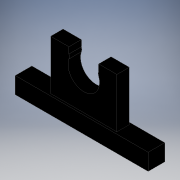
# Autodesk Inventor part: OpticalDeviceLensHolder
Saved by Autodesk Inventor 2017 (Build 210142000, 142)
## iProperties
Created: 2019-04-03
Part Number: OpticalDeviceLensHolder
Material: Generic
Document SubType Name: Modeling
Designer: Sharat
Density: 1 g/cm^3
Appearance: Anodized - Black
Author: Sharat
Autodesk Inventor part; units mm, degrees
ref_plane "YZ Plane" through (0, 0, 0) normal (1, 0, 0) x (0, 1, 0)
ref_plane "XZ Plane" through (0, 0, 0) normal (0, 1, 0) x (-1, 0, 0)
ref_plane "XY Plane" through (0, 0, 0) normal (0, 0, 1) x (1, 0, 0)
sketch "Sketch1" plane through (0, 0, 0) normal (0, 1, 0) x (-1, 0, 0)
  line L0 (0, 0) -> (-160.48, 0)
  line L1 (-160.48, 0) -> (-160.48, -20)
  line L2 (-160.48, -20) -> (0, -20)
  line L3 (0, -20) -> (0, 0)
  dimension "d0" = 160.48
  dimension "d1" = 20
  constraints: 8 end point, 2 parallel, 1 horizontal, 1 perpendicular
  measures "d0" distance of L1.end L2.end
  measures "d1" distance of L2.end L0.start
extrude "Extrusion1" add sketch "Sketch1" along normal blind 20
sketch "Sketch2" plane through (0, 20, 0) normal (0, 1, 0) x (1, 0, 0)
  line L0 (40.24, 17.5) -> (120.24, 17.5)
  line L1 (120.24, 17.5) -> (120.24, 2.5)
  line L2 (120.24, 2.5) -> (40.24, 2.5)
  line L3 (40.24, 2.5) -> (40.24, 17.5)
  line L4 (160.48, 20) -> (0, 20) projected
  line L5 (160.48, 0) -> (160.48, 20) projected
  point P0 (0, 0)
  point P1 (80.24, 17.5)
  point P2 (80.24, 20)
  point P3 (160.48, 10)
  point P4 (120.24, 10)
  dimension "d4" = 80
  dimension "d5" = 15
  constraints: 8 end point, 4 midpoint, 2 parallel, 1 horizontal, 1 horizontal alignment, 1 perpendicular, 1 vertical alignment
  measures "d4" distance of L0.start L0.end
  measures "d5" distance of L0.end L1.end
extrude "Extrusion2" add sketch "Sketch2" along normal blind 60
sketch "Sketch3" plane through (40.24, 20, -2.5) normal (0, 0, 1) x (1, 0, 0)
  circle A0 centre (40, 41) radius 19
  line L0 (0, 60) -> (80, 60) projected
  point P0 (-40.24, -20)
  point P1 (40, 60)
  dimension "d8" = 38
  dimension "d9" = 19
  constraints: 1 centre point, 1 midpoint, 1 vertical alignment
  measures "d8" diameter of A0
  measures "d9" distance from line of L0 A0.centre
extrude "Extrusion3" cut sketch "Sketch3" against normal blind 15
sketch "Sketch4" plane through (40.24, 20, -2.5) normal (0, 0, 1) x (1, 0, 0)
  line L0 (22.0399, 60) -> (22.0399, 52.4283)
  line L1 (22.0399, 52.4283) -> (24.8213, 52.4283)
  circle A0 centre (40, 41) radius 19 projected
  line L2 (40, 60) -> (22.0399, 60)
  arc A1 (40, 60) -> (24.8213, 52.4283) centre (40, 41) ccw
  point P0 (-40.24, -20)
  dimension "d12" = 7.5717
  dimension "d13" = 17.9601
  constraints: 6 end point, 3 point on circle, 1 centre point, 1 concentric, 1 parallel, 1 perpendicular, 1 tangent, 1 vertical
  measures "d12" distance between parallel lines of L2 L1
  measures "d13" distance from line of L2.start L0
extrude "Extrusion4" cut sketch "Sketch4" against normal blind 15 contours L2 A0 L1 L0
sketch "Sketch5" plane through (40.24, 20, -2.5) normal (0, 0, 1) x (1, 0, 0)
  arc A0 (24.8213, 52.4283) -> (40, 60) centre (40, 41) ccw projected
  line L0 (55.1787, 52.4283) -> (57.9578, 52.4283)
  line L1 (57.9578, 52.4283) -> (57.9578, 60)
  line L2 (57.9578, 60) -> (40, 60)
  line L3 (80, 60) -> (40, 60) projected
  arc A1 (55.1787, 52.4283) -> (40, 60) centre (40, 41) ccw
  point P0 (-40.24, -20)
  dimension "d16" = 17.9578
  dimension "d17" = 2.7791
  dimension "d18" = 7.5717
  constraints: 6 end point, 3 point on circle, 2 perpendicular, 1 centre point, 1 concentric, 1 horizontal, 1 tangent
  measures "d16" distance of L1.end L2.end
  measures "d17" distance of L0.start L0.end
  measures "d18" distance between parallel lines of L0 L2
extrude "Extrusion5" cut sketch "Sketch5" against normal blind 15
fillet "Fillet1" radius 7.62 1 edges at (95.4187, 72.4283, -10)
fillet "Fillet2" radius 7.62 1 edges at (65.0613, 72.4283, -10)
body "Solid1"
